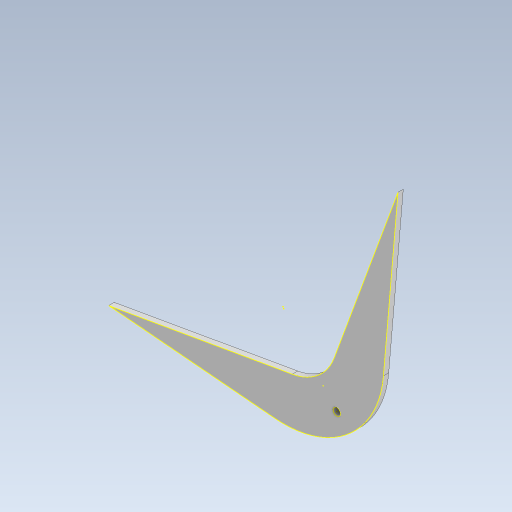
# Autodesk Inventor part: sus_1
Saved by Autodesk Inventor 2023 (Build 270158000, 158)
## iProperties
Created: 2023-06-07
Part Number: sus_1
Material: 一般
Document SubType Name: Modeling
Designer: JOU
Density: 1 g/cm^3
Appearance: 預設
Author: JOU
Autodesk Inventor part; units mm, degrees
ref_plane "YZ Plane" through (0, 0, 0) normal (1, 0, 0) x (0, 1, 0)
ref_plane "XZ Plane" through (0, 0, 0) normal (0, 1, 0) x (-1, 0, 0)
ref_plane "XY Plane" through (0, 0, 0) normal (0, 0, 1) x (1, 0, 0)
sketch "草圖1" plane through (0, 0, 0) normal (0, 0, 1) x (1, 0, 0)
  arc A0 (-17.0574, -3.0077) -> (5.924, 16.276) centre (-22.2668, 26.5366) ccw
  line L0 (5.924, 16.276) -> (41.0424, 112.7631)
  line L1 (-118.1769, -20.8378) -> (-17.0574, -3.0077)
  line L2 (-118.1769, -20.8378) -> (-26.5575, -28.8534)
  arc A1 (-26.5575, -28.8534) -> (33.0268, 21.1437) centre (-21.764, 25.9373) ccw
  line L3 (33.0268, 21.1437) -> (41.0424, 112.7631)
  circle A2 centre (7.3253, -8.7299) radius 2
  point P0 (0, 0)
  dimension "d0" = 55
  dimension "d1" = 4
  dimension "d2" = 23
  dimension "d3" = 23
  constraints: 8 end point, 4 point on circle, 3 centre point, 2 perpendicular, 2 tangent, 8 other
  measures "d0" radius of A1
  measures "d1" diameter of A2
  measures "d2" distance from line of L3 A2.centre
  measures "d3" distance from line of L2 A2.centre
extrude "擠出1" add sketch "草圖1" along normal blind 3
sketch "草圖2" plane through (0, 0, 3) normal (0, 0, 1) x (1, 0, 0)
  arc A0 (-26.5575, -28.8534) -> (33.0268, 21.1437) centre (-21.764, 25.9373) ccw projected
  line L0 (33.0268, 21.1437) -> (41.0424, 112.7631) projected
  line L1 (41.0424, 112.7631) -> (5.924, 16.276) projected
  arc A1 (-17.0574, -3.0077) -> (5.924, 16.276) centre (-22.2668, 26.5366) ccw projected
  line L2 (-17.0574, -3.0077) -> (-118.1769, -20.8378) projected
  line L3 (-118.1769, -20.8378) -> (-26.5575, -28.8534) projected
  circle A2 centre (7.3253, -8.7299) radius 2 projected
  point P0 (0, 0)
equation "\"d3\" = d2"
